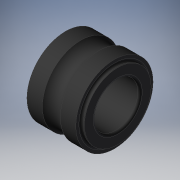
# Autodesk Inventor part: SKF_W 624 R_PART1
Saved by Autodesk Inventor 2019 (Build 230136000, 136)
## iProperties
Created: 2022-09-09
Part Number: SKF_W 624 R_PART1
Material: Generic
Catalog Web Link: www.cadenas.de
Description: -Deep groove ball bearings
Vendor: SKF
Document SubType Name: Modeling
Designer: psAdmin
Manufacturer: SKF
Mass: 3 g
Surface Area: 2.16794 cm^2
Volume: 0.113806 cm^3
Density: 1 g/cm^3
Appearance: PSOLRGB-175-175-175
Category: PARTsolutions
Company: SKF
Title: SKF_W 624 R_PART1
Author: Cadenas PARTsolutions
Comments: Deep groove ball bearings
PSOL_IDENT_0: {$CADENAS_DATA/23d-libs/skf/bearings_units_and_housings/ball_bearings/deep_groove_ball_bearings/bb1_
PSOL_IDENT_1: 001_101.prj},201 {VTYP=3D},{NB=SKF_W 624 R_PART1},{LINA=SKF_W 624 R_PART1},{NN=BB1_001_101_PART1},{N
PSOL_IDENT_2: OPRJ=TRUE},{DATE=04.08.2022 15:25:15},{GEOMDATE=04.07.2022 10:54:51},{VERSION=},{LINEID=21510},{WBVA
PSOL_IDENT_3: R=},{WBNUMERIC=}  {NB=SKF_W 624 R_PART1},{LINA=SKF_W 624 R_PART1},{KT=DUMMY},{DESIGNATION=W 624 R},{
PSOL_IDENT_4: R12=0.20},{DD=4.000},{D=13.000},{B=5.000},{C=},{CX=},{CXX=1},{CA=1.000},{XXVARIANT=Flanged outer rin
PSOL_IDENT_5: g},{XXDESIGN=Single row stainless steel},{XXSEALING=No seals},{DESIGN=dgbbwr2zs},{DESIGNIR=dgbbwr2zs
PSOL_IDENT_6: },{VARIANT=Flanged outer ring},{DD1=6.95},{DD2=6},{DD2X=},{DD2A=6.00},{D1=10.45},{D1X=0.00},{D2=11.3
PSOL_IDENT_7: 5},{D2A=11.35},{D3=15},{D3X=},{D3A=15.000},{D4=},{HH=0.000},{BB=0.000},{BBX=},{BBA=0.000},{FF=},{R0M
PSOL_IDENT_8: AX=0.000},{R0=0.000},{PITCH=8.70},{DW=2.381},{DDAMIN=5.600},{DDAMAX=0.000},{DDBMIN=0.000},{DDBMAX=0.
PSOL_IDENT_9: 000},{DBMIN=0.000},{DAMAX=0.000},{BBAMIN=0.000},{CAMAX=0.000},{RAMAX=0.200},{LOAD1=0.741},{LOAD2=0.2
PSOL_IDENT_10: 50},{LOAD3=0.011},{SPEED1=110000},{SPEED2=70000},{KR=0.030},{F0=6.400},{Z=7},{II=1},{MASS=0.003},{BE
PSOL_IDENT_11: ARING=W 624 R},{RING=},{HELP=1.275},{HELP2=0.825},{DD1ALG=3.475},{YALG=3.475},{PITCH1=8.700},{DW1=2.
PSOL_IDENT_12: 381},{YALG1=5.225},{HALG1=1.275},{SH=3.000},{CU=0.524},{HALG=1.475},{B1=-2.82145},{SHIELDHELP=1},{D4
PSOL_IDENT_13: A=0.000},{FFA=0.000},{RS1=},{HELP3=0}
NB: SKF_W 624 R_PART1
NT: Deep groove ball bearings
NBSYN: SKF_$DESIGNATION._PART1
LINA: SKF_W 624 R_PART1
CATALOG: SKF
DESIGNATION: W 624 R
R12: 0.2
DD: 4
D: 13
B: 5
XXVARIANT: Flanged outer ring
XXDESIGN: Single row stainless steel
XXSEALING: No seals
DD2: 6
D2: 11.35
LOAD1: 0.741
LOAD2: 0.25
LOAD3: 0.011
SPEED1: 110000
SPEED2: 70000
BEARING: W 624 R
SUPPLIER: SKF
ARTICLENO: SKF_W 624 R_PART1
BOMINFO: SKF_W 624 R_PART1
CREATOR: CADENAS GmbH
Autodesk Inventor part; units mm, degrees
ref_plane "YZ Plane" through (0, 0, 0) normal (1, 0, 0) x (0, 1, 0)
ref_plane "XZ Plane" through (0, 0, 0) normal (0, 1, 0) x (-1, 0, 0)
ref_plane "XY Plane" through (0, 0, 0) normal (0, 0, 1) x (1, 0, 0)
sketch "Sketch_40" plane through (0, 0, 0) normal (0, 0, 1) x (1, 0, 0)
  line L0 (2.5, 0) -> (-2.5, 0)
  line L1 (0, 3.425) -> (0, 2.2)
  arc A0 (0, 2.2) -> (0.2, 2) centre (0.2, 2.2) ccw
  line L2 (0.2, 2) -> (4.8, 2)
  arc A1 (4.8, 2) -> (5, 2.2) centre (4.8, 2.2) ccw
  line L3 (5, 2.2) -> (5, 3.425)
  arc A2 (5, 3.425) -> (4.95, 3.475) centre (4.95, 3.425) ccw
  line L4 (4.95, 3.475) -> (3.3073, 3.475)
  arc A3 (1.6927, 3.475) -> (3.3073, 3.475) centre (2.5, 4.35) ccw
  line L5 (1.6927, 3.475) -> (0.05, 3.475)
  arc A4 (0.05, 3.475) -> (0, 3.425) centre (0.05, 3.425) ccw
  constraints: 12 end point, 10 point on circle, 5 centre point
revolve "Revolution1" add sketch "Sketch_40" angle 360 about axis through (2.5, 0, 0) along (1, 0, 0)
sketch "Sketch_42" plane through (0, 0, 0) normal (0, 0, 1) x (1, 0, 0)
  line L0 (2.5, 0) -> (-2.5, 0)
  line L1 (0, 7.35) -> (0, 3)
  line L2 (0, 3) -> (0.1, 3)
  arc A0 (0.1, 3) -> (0.3, 3.2) centre (0.1, 3.2) ccw
  line L3 (0.3, 3.2) -> (0.3, 7.15)
  line L4 (0.3, 7.15) -> (4.7, 7.15)
  line L5 (4.7, 7.15) -> (4.7, 3.2)
  arc A1 (4.7, 3.2) -> (4.9, 3) centre (4.9, 3.2) ccw
  line L6 (4.9, 3) -> (5, 3)
  line L7 (5, 3) -> (5, 7.35)
  line L8 (5, 7.35) -> (0, 7.35)
  constraints: 18 end point, 4 point on circle, 2 centre point
revolve "Revolution2" cut sketch "Sketch_42" angle 360 about axis through (2.5, 0, 0) along (1, 0, 0)
body "Solid1"
